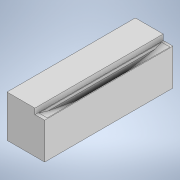
# Autodesk Inventor part: ball collector
Saved by Autodesk Inventor 2020 (Build 240168000, 168)
## iProperties
Created: 2021-03-06
Part Number: ball collector
Material: Generic
Document SubType Name: Modeling
Designer: Harry
Density: 1 g/cm^3
Appearance: Default
Author: Harry
Autodesk Inventor part; units mm, degrees
ref_plane "YZ Plane" through (0, 0, 0) normal (1, 0, 0) x (0, 1, 0)
ref_plane "XZ Plane" through (0, 0, 0) normal (0, 1, 0) x (-1, 0, 0)
ref_plane "XY Plane" through (0, 0, 0) normal (0, 0, 1) x (1, 0, 0)
sketch "Sketch1" plane through (0, 0, 0) normal (0, 1, 0) x (-1, 0, 0)
  line L0 (-50, -230) -> (50, -230)
  line L1 (50, -230) -> (50, 230)
  line L2 (50, 230) -> (-50, 230)
  line L3 (-50, 230) -> (-50, -230)
  line L4 (-50, -230) -> (50, 230) construction
  line L5 (50, -230) -> (-50, 230) construction
  point P0 (0, 0)
  dimension "d0" = 100
  dimension "d1" = 460
  constraints: 12 end point, 2 midpoint, 2 parallel, 1 horizontal, 1 perpendicular
  measures "d0" distance of L2.end L1.end
  measures "d1" distance of L1.end L0.end
extrude "Extrusion1" add sketch "Sketch1" along normal blind 150
sketch "Sketch2" plane through (50, 0, 230) normal (1, 0, 0) x (0, 0, -1)
  line L0 (0, 0) -> (0, 150) projected
  line L1 (460, 0) -> (460, 150) projected
  line L2 (0, 0) -> (460, 0)
  line L3 (460, 0) -> (460, 130)
  line L4 (460, 130) -> (0, 130)
  line L5 (0, 130) -> (0, 0)
  point P0 (230, 0)
  dimension "d4" = 130
  constraints: 8 end point, 2 parallel, 1 horizontal, 1 perpendicular, 1 point on line
  measures "d4" distance of L3.end L2.end
extrude "Extrusion2" add sketch "Sketch2" along normal blind 35
sketch "Sketch3" plane through (50, 130, 230) normal (0, 1, 0) x (1, 0, 0)
  line L0 (-100, 0) -> (35, 0) projected
  line L1 (-100, 460) -> (35, 460) projected
  line L2 (-0.5456, 0) -> (35, 460) construction
  line L3 (0, 0) -> (0, 460) projected
  line L4 (0, 460) -> (35, 0) construction
  line L5 (27.3646, 241.7789) -> (7.3646, 241.7789)
  line L6 (7.3646, 241.7789) -> (7.3646, 221.7789)
  line L7 (7.3646, 221.7789) -> (27.3646, 221.7789)
  line L8 (27.3646, 221.7789) -> (27.3646, 241.7789)
  line L9 (27.3646, 241.7789) -> (7.3646, 221.7789) construction
  line L10 (7.3646, 241.7789) -> (27.3646, 221.7789) construction
  point P0 (-50, 230)
  point P1 (17.3646, 231.7789)
  dimension "d7" = 20
  dimension "d8" = 20
  constraints: 16 end point, 3 point on line, 2 midpoint, 2 parallel, 1 horizontal, 1 perpendicular
  measures "d7" distance of L7.end L6.end
  measures "d8" distance of L6.end L5.end
extrude "Extrusion3" cut sketch "Sketch3" against normal blind 165
chamfer "Chamfer1" distance 210 angle 10 1 edges at (67.3646, 130, 8.2211) measured on face at (67.3646, 130, 8.7211)
chamfer "Chamfer2" distance 210 angle 10 1 edges at (67.3646, 130, -11.7789) measured on face at (67.3646, 130, -12.2789)
chamfer "Chamfer3" distance 5 angle 45 3 edges at (57.3646, 130, -116.7789) (57.3646, 130, -1.7789) (57.3646, 130, 113.2211)
chamfer "Chamfer4" distance 5 angle 45 3 edges at (77.3646, 130, 113.2211) (77.3646, 130, -1.7789) (77.3646, 130, -116.7789)
body "Solid1"
